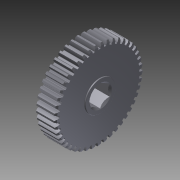
# Autodesk Inventor part: AM-0129 Large Final Gear 45T
Saved by Autodesk Inventor 2014 SP1 (Build 180222100, 222)
## iProperties
Shininess: 64.0
Length Units: 11272
Angle Units: 11279
Time Units: 11290
Mass Units: 11286
Length Display Precision: 3
Angle Display Precision: 2
Category: FIRST Robotics Components
Manager: Ed Sparks
Company: FIRST CAD Library
Created: 2003-12-13
Part Number: AM-0129 Large Final Gear 45T
Project: FIRST
Material: Steel, High Strength Low Alloy
Document SubType Name: Modeling
Designer: Ed Sparks
Engineer: Ed Sparks
Catalog Web Link: www.firstcadlibrary.com
Density: 7.84 g/cm^3
Mass: 255.147 g
Surface Area: 103.524 cm^2
Volume: 32.5442 cm^3
Appearance: Steel
Density: 7.84
Volumn: 6.736982259993864
Area: 35.592573078640946
PropertySet Name: Model Information
Control State: 0
Master: False
Checked Out: False
Title: Gear
Subject: Robot Component
Author: Ed Sparks
Keywords: FIRST
Autodesk Inventor part; units mm, degrees
ref_plane "YZ Plane" through (0, 0, 0) normal (1, 0, 0) x (0, 1, 0)
ref_plane "XZ Plane" through (0, 0, 0) normal (0, 1, 0) x (-1, 0, 0)
ref_plane "XY Plane" through (0, 0, 0) normal (0, 0, 1) x (1, 0, 0)
sketch "Sketch2" plane through (6.7691, 0, 0) normal (1, 0, 0) x (0, 0, -1)
  circle A0 centre (0, 0) radius 27.6648 construction
  arc A1 (1.4999, 29.8073) -> (-1.4999, 29.8073) centre (0, 0) ccw
  line L0 (0.9975, 28.5576) -> (7.8574, 26.5255) construction
  line L1 (0, 0) -> (0, 25.7198) construction
  circle A2 centre (0, 0) radius 28.575 projected
  arc A3 (1.4999, 29.8073) -> (0.7359, 27.2128) centre (7.8574, 26.5255) ccw
  arc A4 (-0.7359, 27.2128) -> (-1.4999, 29.8073) centre (-7.8574, 26.5255) ccw
  arc A5 (0.4786, 26.9833) -> (-0.4786, 26.9833) centre (0, 0) ccw
  line L2 (0, 0) -> (0, 42.0936) construction
  circle A6 centre (0, 0) radius 6.35 projected
  circle A7 centre (0, 0) radius 28.575 construction
  line L3 (-7.8574, 26.5255) -> (-0.9975, 28.5576) construction
  arc A8 (-0.7359, 27.2128) -> (-0.4786, 26.9833) centre (-0.4831, 27.2372) ccw
  arc A9 (0.4786, 26.9833) -> (0.7359, 27.2128) centre (0.4831, 27.2372) ccw
  dimension "d24" = 55.3296
  dimension "Root_Radius" = 26.9875
  dimension "d104" = 29.845
  dimension "Pitch_Diameter" = 57.15
  dimension "Tooth_Width" = 1.9949
  dimension "Root_Fillet" = 0.254
  dimension "d112" = 0.254
  constraints: 16 point on circle, 8 end point, 7 centre point, 6 coincident, 4 tangent, 1 point on line, 1 vertical, 6 other
  measures "Root_Radius" radius of A5
  measures "d104" radius of A1
  measures "Pitch_Diameter" diameter of A7
  measures "Tooth_Width" distance of L0.start L3.end
  measures "Root_Fillet" radius of A8
  measures "d112" radius of A9
sketch "Sketch1" plane through (0, 0, 0) normal (0, 0, 1) x (1, 0, 0)
  line L0 (6.7691, 6.35) -> (6.7691, 28.575)
  line L1 (6.0359, 29.845) -> (-6.0359, 29.845)
  line L2 (-6.7691, 28.575) -> (-6.7691, 6.35)
  line L3 (-6.7691, 6.35) -> (6.7691, 6.35)
  line L4 (6.7691, 28.575) -> (6.0359, 29.845)
  line L5 (-6.7691, 28.575) -> (-6.0359, 29.845)
  line L6 (-5.715, 0) -> (7.62, 0) projected
  line L7 (0, 0) -> (0, 27.4224) construction
  point P0 (0, 6.35)
  dimension "Bore_Radius" = 6.35
  dimension "Outside_Radius" = 29.845
  dimension "d77" = 28.575
  dimension "d108" = 30
  dimension "d109" = 30
  dimension "d110" = 13.5382
  constraints: 14 end point, 3 vertical, 2 perpendicular, 1 coincident, 1 horizontal alignment, 1 midpoint, 1 point on line, 2 other
  measures "Bore_Radius" distance from line of point (0, 0) L3
  measures "Outside_Radius" distance from line of point (0, 0) L1
  measures "d77" distance from line of L6 L0.end
  measures "d108" angle of L5 L2
  measures "d109" angle of L4 L0
  measures "d110" distance of L2.end L0.start
revolve "Gear Blank" add sketch "Sketch1" angle 360 about axis through (-10, 0, 0) along (1, 0, 0)
extrude "Tooth Profile" cut sketch "Sketch2" against normal through all contours A3 A2 A4 A1 | A3 A9 A5 A8 A4 A2 picked at (-0.1108, 27.9686)
pattern_circular "Circular Pattern" count 45 over 360 about axis through (0, 0, 0) along (1, 0, 0) of "Tooth Profile"
chamfer "Bore Chamfer Interior" [suppressed]
sketch "Sketch3" plane through (6.7691, 26.5255, -7.8574) normal (1, 0, 0) x (0, -0.19092, -0.9816056)
  circle A0 centre (-2.6486, -27.5377) radius 6.35 projected
  arc A1 (5.9188, -0.0546) -> (3.9761, 0.4252) centre (-2.6486, -27.5377) ccw projected
  circle A2 centre (-2.6486, -27.5377) radius 10.16
  dimension "d31" = 20.32
  constraints: 1 centre point, 1 coincident, 1 other
  measures "d31" diameter of A2
extrude "Hub" add sketch "Sketch3" along normal blind 0.762
fillet "Hub Fillet" radius 0.254 2 edges at (6.7691, 1.9397, 9.9731) (7.5311, 1.9397, 9.9731)
chamfer "Bore Chamfer Exterior" distance 1.27 angle 45 1 edges at (-6.7691, -6.35, 0)
chamfer "Bore Chamfer on Hub" distance 1.27 angle 45 1 edges at (7.5311, 1.2123, 6.2332)
sketch "Sketch5" plane through (0, 0, 0) normal (1, 0, 0) x (0, 1, 0)
  line L0 (3.6662, 6.35) -> (7.3323, 0)
  line L1 (7.3323, 0) -> (3.6662, -6.35)
  line L2 (3.6662, -6.35) -> (-3.6662, -6.35)
  line L3 (-3.6662, -6.35) -> (-7.3323, 0)
  line L4 (-7.3323, 0) -> (-3.6662, 6.35)
  line L5 (-3.6662, 6.35) -> (3.6662, 6.35)
  point P0 (0, 0)
  dimension "d78" = 12.7
  constraints: 12 end point, 1 horizontal, 12 other
  measures "d78" distance between parallel lines of L1 L4
extrude "Hex Broach" cut sketch "Sketch5" along normal through all both and the other way through all
sketch "Sketch16" plane through (0, 0, 0) normal (1, 0, 0) x (0, 1, 0)
  line L0 (7.5406, -1.1906) -> (5.1594, -1.1906)
  line L1 (5.1594, -1.1906) -> (5.1594, 1.1906)
  line L2 (5.1594, 1.1906) -> (7.5406, 1.1906)
  line L3 (7.5406, 1.1906) -> (7.5406, -1.1906)
  line L4 (0, 0) -> (9.5781, 0) construction
  line L5 (0, 0) -> (0, 8.8774) construction
  dimension "d117" = 2.3813
  dimension "d118" = 5.1594
  constraints: 12 end point, 3 horizontal, 2 parallel, 2 perpendicular, 2 vertical, 1 other
  measures "d117" distance of L2.end L0.start
  measures "d118" distance between parallel lines of L5 L1
extrude "Key" [suppressed]
equation "\"d31\" = Hub_Diameter"
equation "\"d32\" = Hub_Thickness"
equation "\"Bore_Radius\" = 0.5 * Bore"
equation "\"Bore\" = 12.7"
equation "\"Pressure_Angle\" = 14.5deg"
equation "\"Hub_Diameter\" = 20.32"
equation "\"Hub_Thickness\" = 0.762"
equation "\"Key_Size\" = 2.38125"
equation "\"Bore_Chamfer\" = 1.27"
equation "\"Face_Width\" = 13.5382"
equation "\"Tooth_Chamfer\" = 30deg"
body "Solid1"
